Autodesk Fusion 360 part; units mm, degrees
(part 31 of 40)
  spline S99 degree 5 poles (217.8271, 89.2315) (217.8299, 89.2007) (217.8349, 89.1391) (217.8398, 89.0467) (217.8417, 88.9234) (217.8376, 88.769) (217.8289, 88.6144) (217.8174, 88.4597) (217.8043, 88.305) (217.7903, 88.1502) (217.7751, 87.9955) (217.7585, 87.8407) (217.74, 87.686) (217.7191, 87.5312) (217.6961, 87.3765) (217.671, 87.2218) (217.6441, 87.0671) (217.6158, 86.9125) (217.5862, 86.7579) (217.5553, 86.6034) (217.5233, 86.4489) (217.4899, 86.2945) (217.4552, 86.1402) (217.4191, 85.986) (217.3817, 85.8318) (217.3429, 85.6778) (217.3029, 85.5238) (217.2617, 85.3699) (217.2193, 85.2161) (217.1759, 85.0624) (217.1313, 84.9088) (217.0856, 84.7553) (217.0388, 84.602) (216.9909, 84.4487) (216.9419, 84.2956) (216.8919, 84.1426) (216.8407, 83.9897) (216.7886, 83.8369) (216.7355, 83.6842) (216.6813, 83.5317) (216.6262, 83.3794) (216.57, 83.2271) (216.513, 83.075) (216.4549, 82.923) (216.3959, 82.7712) (216.3359, 82.6196) (216.275, 82.468) (216.2132, 82.3167) (216.1505, 82.1655) (216.0868, 82.0144) (216.0223, 81.8635) (215.9569, 81.7128) (215.8905, 81.5622) (215.8233, 81.4118) (215.7553, 81.2616) (215.6863, 81.1115) (215.6166, 80.9616) (215.5459, 80.8119) (215.4745, 80.6624) (215.4021, 80.513) (215.329, 80.3638) (215.255, 80.2148) (215.1802, 80.066) (215.1046, 79.9174) (215.0282, 79.7689) (214.951, 79.6207) (214.873, 79.4726) (214.7942, 79.3248) (214.7146, 79.1771) (214.6343, 79.0297) (214.5531, 78.8824) (214.4876, 78.7648) (214.4381, 78.6766) (214.4049, 78.6179) (214.3883, 78.5885) knots 0 0 0 0 0 0 0.01428571 0.02857143 0.04285714 0.05714286 0.07142857 0.08571429 0.1 0.11428571 0.12857143 0.14285714 0.15714286 0.17142857 0.18571429 0.2 0.21428571 0.22857143 0.24285714 0.25714286 0.27142857 0.28571429 0.3 0.31428571 0.32857143 0.34285714 0.35714286 0.37142857 0.38571429 0.4 0.41428571 0.42857143 0.44285714 0.45714286 0.47142857 0.48571429 0.5 0.51428571 0.52857143 0.54285714 0.55714286 0.57142857 0.58571429 0.6 0.61428571 0.62857143 0.64285714 0.65714286 0.67142857 0.68571429 0.7 0.71428571 0.72857143 0.74285714 0.75714286 0.77142857 0.78571429 0.8 0.81428571 0.82857143 0.84285714 0.85714286 0.87142857 0.88571429 0.9 0.91428571 0.92857143 0.94285714 0.95714286 0.97142857 0.98571429 1 1 1 1 1 1
  line L7434 (217.8271, 89.2315) -> (217.8299, 89.2007) construction
  line L7435 (217.8299, 89.2007) -> (217.8349, 89.1391) construction
  line L7436 (217.8349, 89.1391) -> (217.8398, 89.0467) construction
  line L7437 (217.8398, 89.0467) -> (217.8417, 88.9234) construction
  line L7438 (217.8417, 88.9234) -> (217.8376, 88.769) construction
  line L7439 (217.8376, 88.769) -> (217.8289, 88.6144) construction
  line L7440 (217.8289, 88.6144) -> (217.8174, 88.4597) construction
  line L7441 (217.8174, 88.4597) -> (217.8043, 88.305) construction
  line L7442 (217.8043, 88.305) -> (217.7903, 88.1502) construction
  line L7443 (217.7903, 88.1502) -> (217.7751, 87.9955) construction
  line L7444 (217.7751, 87.9955) -> (217.7585, 87.8407) construction
  line L7445 (217.7585, 87.8407) -> (217.74, 87.686) construction
  line L7446 (217.74, 87.686) -> (217.7191, 87.5312) construction
  line L7447 (217.7191, 87.5312) -> (217.6961, 87.3765) construction
  line L7448 (217.6961, 87.3765) -> (217.671, 87.2218) construction
  line L7449 (217.671, 87.2218) -> (217.6441, 87.0671) construction
  line L7450 (217.6441, 87.0671) -> (217.6158, 86.9125) construction
  line L7451 (217.6158, 86.9125) -> (217.5862, 86.7579) construction
  line L7452 (217.5862, 86.7579) -> (217.5553, 86.6034) construction
  line L7453 (217.5553, 86.6034) -> (217.5233, 86.4489) construction
  line L7454 (217.5233, 86.4489) -> (217.4899, 86.2945) construction
  line L7455 (217.4899, 86.2945) -> (217.4552, 86.1402) construction
  line L7456 (217.4552, 86.1402) -> (217.4191, 85.986) construction
  line L7457 (217.4191, 85.986) -> (217.3817, 85.8318) construction
  line L7458 (217.3817, 85.8318) -> (217.3429, 85.6778) construction
  line L7459 (217.3429, 85.6778) -> (217.3029, 85.5238) construction
  line L7460 (217.3029, 85.5238) -> (217.2617, 85.3699) construction
  line L7461 (217.2617, 85.3699) -> (217.2193, 85.2161) construction
  line L7462 (217.2193, 85.2161) -> (217.1759, 85.0624) construction
  line L7463 (217.1759, 85.0624) -> (217.1313, 84.9088) construction
  line L7464 (217.1313, 84.9088) -> (217.0856, 84.7553) construction
  line L7465 (217.0856, 84.7553) -> (217.0388, 84.602) construction
  line L7466 (217.0388, 84.602) -> (216.9909, 84.4487) construction
  line L7467 (216.9909, 84.4487) -> (216.9419, 84.2956) construction
  line L7468 (216.9419, 84.2956) -> (216.8919, 84.1426) construction
  line L7469 (216.8919, 84.1426) -> (216.8407, 83.9897) construction
  line L7470 (216.8407, 83.9897) -> (216.7886, 83.8369) construction
  line L7471 (216.7886, 83.8369) -> (216.7355, 83.6842) construction
  line L7472 (216.7355, 83.6842) -> (216.6813, 83.5317) construction
  line L7473 (216.6813, 83.5317) -> (216.6262, 83.3794) construction
  line L7474 (216.6262, 83.3794) -> (216.57, 83.2271) construction
  line L7475 (216.57, 83.2271) -> (216.513, 83.075) construction
  line L7476 (216.513, 83.075) -> (216.4549, 82.923) construction
  line L7477 (216.4549, 82.923) -> (216.3959, 82.7712) construction
  line L7478 (216.3959, 82.7712) -> (216.3359, 82.6196) construction
  line L7479 (216.3359, 82.6196) -> (216.275, 82.468) construction
  line L7480 (216.275, 82.468) -> (216.2132, 82.3167) construction
  line L7481 (216.2132, 82.3167) -> (216.1505, 82.1655) construction
  line L7482 (216.1505, 82.1655) -> (216.0868, 82.0144) construction
  line L7483 (216.0868, 82.0144) -> (216.0223, 81.8635) construction
  line L7484 (216.0223, 81.8635) -> (215.9569, 81.7128) construction
  line L7485 (215.9569, 81.7128) -> (215.8905, 81.5622) construction
  line L7486 (215.8905, 81.5622) -> (215.8233, 81.4118) construction
  line L7487 (215.8233, 81.4118) -> (215.7553, 81.2616) construction
  line L7488 (215.7553, 81.2616) -> (215.6863, 81.1115) construction
  line L7489 (215.6863, 81.1115) -> (215.6166, 80.9616) construction
  line L7490 (215.6166, 80.9616) -> (215.5459, 80.8119) construction
  line L7491 (215.5459, 80.8119) -> (215.4745, 80.6624) construction
  line L7492 (215.4745, 80.6624) -> (215.4021, 80.513) construction
  line L7493 (215.4021, 80.513) -> (215.329, 80.3638) construction
  line L7494 (215.329, 80.3638) -> (215.255, 80.2148) construction
  line L7495 (215.255, 80.2148) -> (215.1802, 80.066) construction
  line L7496 (215.1802, 80.066) -> (215.1046, 79.9174) construction
  line L7497 (215.1046, 79.9174) -> (215.0282, 79.7689) construction
  line L7498 (215.0282, 79.7689) -> (214.951, 79.6207) construction
  line L7499 (214.951, 79.6207) -> (214.873, 79.4726) construction
  line L7500 (214.873, 79.4726) -> (214.7942, 79.3248) construction
  line L7501 (214.7942, 79.3248) -> (214.7146, 79.1771) construction
  line L7502 (214.7146, 79.1771) -> (214.6343, 79.0297) construction
  line L7503 (214.6343, 79.0297) -> (214.5531, 78.8824) construction
  line L7504 (214.5531, 78.8824) -> (214.4876, 78.7648) construction
  line L7505 (214.4876, 78.7648) -> (214.4381, 78.6766) construction
  line L7506 (214.4381, 78.6766) -> (214.4049, 78.6179) construction
  line L7507 (214.4049, 78.6179) -> (214.3883, 78.5885) construction
  spline S100 degree 5 poles (257.9473, 109.6737) (257.9705, 109.6533) (258.0174, 109.6132) (258.0893, 109.5549) (258.188, 109.4808) (258.3153, 109.3934) (258.4455, 109.3096) (258.5774, 109.228) (258.7102, 109.1476) (258.8437, 109.068) (258.9778, 108.9893) (259.1127, 108.9117) (259.2488, 108.8358) (259.3863, 108.7617) (259.525, 108.6894) (259.6649, 108.6187) (259.8058, 108.5496) (259.9476, 108.4816) (260.0901, 108.4147) (260.2332, 108.3488) (260.377, 108.284) (260.5215, 108.2202) (260.6667, 108.1576) (260.8127, 108.0961) (260.9594, 108.0358) (261.1069, 107.9766) (261.255, 107.9185) (261.4037, 107.8614) (261.553, 107.8053) (261.7029, 107.7501) (261.8534, 107.6959) (262.0044, 107.6426) (262.156, 107.5903) (262.3081, 107.539) (262.4608, 107.4886) (262.614, 107.4392) (262.7678, 107.3906) (262.922, 107.343) (263.0767, 107.2963) (263.2319, 107.2505) (263.3876, 107.2055) (263.5438, 107.1614) (263.7004, 107.1182) (263.8575, 107.0759) (264.015, 107.0344) (264.1729, 106.9937) (264.3313, 106.9539) (264.4901, 106.915) (264.6493, 106.8769) (264.8089, 106.8396) (264.9689, 106.8031) (265.1293, 106.7674) (265.2901, 106.7326) (265.4513, 106.6985) (265.6129, 106.6653) (265.7748, 106.6328) (265.9371, 106.6012) (266.0997, 106.5703) (266.2627, 106.5403) (266.426, 106.511) (266.5897, 106.4825) (266.7537, 106.4547) (266.9181, 106.4277) (267.0828, 106.4016) (267.2478, 106.3761) (267.4131, 106.3514) (267.5787, 106.3275) (267.7446, 106.3044) (267.9109, 106.282) (268.0774, 106.2603) (268.2442, 106.2394) (268.3779, 106.2233) (268.4783, 106.2115) (268.5453, 106.2038) (268.5789, 106.2) knots 0 0 0 0 0 0 0.01428571 0.02857143 0.04285714 0.05714286 0.07142857 0.08571429 0.1 0.11428571 0.12857143 0.14285714 0.15714286 0.17142857 0.18571429 0.2 0.21428571 0.22857143 0.24285714 0.25714286 0.27142857 0.28571429 0.3 0.31428571 0.32857143 0.34285714 0.35714286 0.37142857 0.38571429 0.4 0.41428571 0.42857143 0.44285714 0.45714286 0.47142857 0.48571429 0.5 0.51428571 0.52857143 0.54285714 0.55714286 0.57142857 0.58571429 0.6 0.61428571 0.62857143 0.64285714 0.65714286 0.67142857 0.68571429 0.7 0.71428571 0.72857143 0.74285714 0.75714286 0.77142857 0.78571429 0.8 0.81428571 0.82857143 0.84285714 0.85714286 0.87142857 0.88571429 0.9 0.91428571 0.92857143 0.94285714 0.95714286 0.97142857 0.98571429 1 1 1 1 1 1
  line L7508 (257.9473, 109.6737) -> (257.9705, 109.6533) construction
  line L7509 (257.9705, 109.6533) -> (258.0174, 109.6132) construction
  line L7510 (258.0174, 109.6132) -> (258.0893, 109.5549) construction
  line L7511 (258.0893, 109.5549) -> (258.188, 109.4808) construction
  line L7512 (258.188, 109.4808) -> (258.3153, 109.3934) construction
  line L7513 (258.3153, 109.3934) -> (258.4455, 109.3096) construction
  line L7514 (258.4455, 109.3096) -> (258.5774, 109.228) construction
  line L7515 (258.5774, 109.228) -> (258.7102, 109.1476) construction
  line L7516 (258.7102, 109.1476) -> (258.8437, 109.068) construction
  line L7517 (258.8437, 109.068) -> (258.9778, 108.9893) construction
  line L7518 (258.9778, 108.9893) -> (259.1127, 108.9117) construction
  line L7519 (259.1127, 108.9117) -> (259.2488, 108.8358) construction
  line L7520 (259.2488, 108.8358) -> (259.3863, 108.7617) construction
  line L7521 (259.3863, 108.7617) -> (259.525, 108.6894) construction
  line L7522 (259.525, 108.6894) -> (259.6649, 108.6187) construction
  line L7523 (259.6649, 108.6187) -> (259.8058, 108.5496) construction
  line L7524 (259.8058, 108.5496) -> (259.9476, 108.4816) construction
  line L7525 (259.9476, 108.4816) -> (260.0901, 108.4147) construction
  line L7526 (260.0901, 108.4147) -> (260.2332, 108.3488) construction
  line L7527 (260.2332, 108.3488) -> (260.377, 108.284) construction
  line L7528 (260.377, 108.284) -> (260.5215, 108.2202) construction
  line L7529 (260.5215, 108.2202) -> (260.6667, 108.1576) construction
  line L7530 (260.6667, 108.1576) -> (260.8127, 108.0961) construction
  line L7531 (260.8127, 108.0961) -> (260.9594, 108.0358) construction
  line L7532 (260.9594, 108.0358) -> (261.1069, 107.9766) construction
  line L7533 (261.1069, 107.9766) -> (261.255, 107.9185) construction
  line L7534 (261.255, 107.9185) -> (261.4037, 107.8614) construction
  line L7535 (261.4037, 107.8614) -> (261.553, 107.8053) construction
  line L7536 (261.553, 107.8053) -> (261.7029, 107.7501) construction
  line L7537 (261.7029, 107.7501) -> (261.8534, 107.6959) construction
  line L7538 (261.8534, 107.6959) -> (262.0044, 107.6426) construction
  line L7539 (262.0044, 107.6426) -> (262.156, 107.5903) construction
  line L7540 (262.156, 107.5903) -> (262.3081, 107.539) construction
  line L7541 (262.3081, 107.539) -> (262.4608, 107.4886) construction
  line L7542 (262.4608, 107.4886) -> (262.614, 107.4392) construction
  line L7543 (262.614, 107.4392) -> (262.7678, 107.3906) construction
  line L7544 (262.7678, 107.3906) -> (262.922, 107.343) construction
  line L7545 (262.922, 107.343) -> (263.0767, 107.2963) construction
  line L7546 (263.0767, 107.2963) -> (263.2319, 107.2505) construction
  line L7547 (263.2319, 107.2505) -> (263.3876, 107.2055) construction
  line L7548 (263.3876, 107.2055) -> (263.5438, 107.1614) construction
  line L7549 (263.5438, 107.1614) -> (263.7004, 107.1182) construction
  line L7550 (263.7004, 107.1182) -> (263.8575, 107.0759) construction
  line L7551 (263.8575, 107.0759) -> (264.015, 107.0344) construction
  line L7552 (264.015, 107.0344) -> (264.1729, 106.9937) construction
  line L7553 (264.1729, 106.9937) -> (264.3313, 106.9539) construction
  line L7554 (264.3313, 106.9539) -> (264.4901, 106.915) construction
  line L7555 (264.4901, 106.915) -> (264.6493, 106.8769) construction
  line L7556 (264.6493, 106.8769) -> (264.8089, 106.8396) construction
  line L7557 (264.8089, 106.8396) -> (264.9689, 106.8031) construction
  line L7558 (264.9689, 106.8031) -> (265.1293, 106.7674) construction
  line L7559 (265.1293, 106.7674) -> (265.2901, 106.7326) construction
  line L7560 (265.2901, 106.7326) -> (265.4513, 106.6985) construction
  line L7561 (265.4513, 106.6985) -> (265.6129, 106.6653) construction
  line L7562 (265.6129, 106.6653) -> (265.7748, 106.6328) construction
  line L7563 (265.7748, 106.6328) -> (265.9371, 106.6012) construction
  line L7564 (265.9371, 106.6012) -> (266.0997, 106.5703) construction
  line L7565 (266.0997, 106.5703) -> (266.2627, 106.5403) construction
  line L7566 (266.2627, 106.5403) -> (266.426, 106.511) construction
  line L7567 (266.426, 106.511) -> (266.5897, 106.4825) construction
  line L7568 (266.5897, 106.4825) -> (266.7537, 106.4547) construction
  line L7569 (266.7537, 106.4547) -> (266.9181, 106.4277) construction
  line L7570 (266.9181, 106.4277) -> (267.0828, 106.4016) construction
  line L7571 (267.0828, 106.4016) -> (267.2478, 106.3761) construction
  line L7572 (267.2478, 106.3761) -> (267.4131, 106.3514) construction
  line L7573 (267.4131, 106.3514) -> (267.5787, 106.3275) construction
  line L7574 (267.5787, 106.3275) -> (267.7446, 106.3044) construction
  line L7575 (267.7446, 106.3044) -> (267.9109, 106.282) construction
  line L7576 (267.9109, 106.282) -> (268.0774, 106.2603) construction
  line L7577 (268.0774, 106.2603) -> (268.2442, 106.2394) construction
  line L7578 (268.2442, 106.2394) -> (268.3779, 106.2233) construction
  line L7579 (268.3779, 106.2233) -> (268.4783, 106.2115) construction
  line L7580 (268.4783, 106.2115) -> (268.5453, 106.2038) construction
  line L7581 (268.5453, 106.2038) -> (268.5789, 106.2) construction
  arc A189 (268.5789, 106.2) -> (271.2313, 109.8508) centre (212.132, 150) ccw
  spline S101 degree 5 poles (171.8057, 104.1847) (171.7853, 104.1615) (171.7452, 104.1146) (171.6869, 104.0427) (171.6128, 103.944) (171.5254, 103.8167) (171.4416, 103.6865) (171.36, 103.5546) (171.2796, 103.4218) (171.2, 103.2883) (171.1213, 103.1542) (171.0437, 103.0193) (170.9678, 102.8832) (170.8937, 102.7457) (170.8214, 102.607) (170.7507, 102.4671) (170.6816, 102.3262) (170.6136, 102.1844) (170.5467, 102.0419) (170.4808, 101.8988) (170.416, 101.755) (170.3522, 101.6105) (170.2896, 101.4653) (170.2281, 101.3193) (170.1678, 101.1726) (170.1086, 101.0251) (170.0505, 100.877) (169.9934, 100.7283) (169.9373, 100.579) (169.8821, 100.4291) (169.8279, 100.2786) (169.7746, 100.1276) (169.7223, 99.976) (169.671, 99.8239) (169.6206, 99.6712) (169.5712, 99.518) (169.5226, 99.3642) (169.475, 99.21) (169.4283, 99.0553) (169.3825, 98.9001) (169.3375, 98.7444) (169.2934, 98.5882) (169.2502, 98.4316) (169.2079, 98.2745) (169.1664, 98.117) (169.1257, 97.9591) (169.0859, 97.8007) (169.047, 97.6419) (169.0089, 97.4827) (168.9716, 97.3231) (168.9351, 97.1631) (168.8994, 97.0027) (168.8646, 96.8419) (168.8305, 96.6807) (168.7973, 96.5191) (168.7648, 96.3572) (168.7332, 96.1949) (168.7023, 96.0323) (168.6723, 95.8693) (168.643, 95.706) (168.6145, 95.5423) (168.5867, 95.3783) (168.5597, 95.2139) (168.5336, 95.0492) (168.5081, 94.8842) (168.4834, 94.7189) (168.4595, 94.5533) (168.4364, 94.3874) (168.414, 94.2211) (168.3923, 94.0546) (168.3714, 93.8878) (168.3553, 93.7541) (168.3435, 93.6537) (168.3358, 93.5867) (168.332, 93.5531) knots 0 0 0 0 0 0 0.01428571 0.02857143 0.04285714 0.05714286 0.07142857 0.08571429 0.1 0.11428571 0.12857143 0.14285714 0.15714286 0.17142857 0.18571429 0.2 0.21428571 0.22857143 0.24285714 0.25714286 0.27142857 0.28571429 0.3 0.31428571 0.32857143 0.34285714 0.35714286 0.37142857 0.38571429 0.4 0.41428571 0.42857143 0.44285714 0.45714286 0.47142857 0.48571429 0.5 0.51428571 0.52857143 0.54285714 0.55714286 0.57142857 0.58571429 0.6 0.61428571 0.62857143 0.64285714 0.65714286 0.67142857 0.68571429 0.7 0.71428571 0.72857143 0.74285714 0.75714286 0.77142857 0.78571429 0.8 0.81428571 0.82857143 0.84285714 0.85714286 0.87142857 0.88571429 0.9 0.91428571 0.92857143 0.94285714 0.95714286 0.97142857 0.98571429 1 1 1 1 1 1
  line L7582 (171.8057, 104.1847) -> (171.7853, 104.1615) construction
  line L7583 (171.7853, 104.1615) -> (171.7452, 104.1146) construction
  line L7584 (171.7452, 104.1146) -> (171.6869, 104.0427) construction
  line L7585 (171.6869, 104.0427) -> (171.6128, 103.944) construction
  line L7586 (171.6128, 103.944) -> (171.5254, 103.8167) construction
  line L7587 (171.5254, 103.8167) -> (171.4416, 103.6865) construction
  line L7588 (171.4416, 103.6865) -> (171.36, 103.5546) construction
  line L7589 (171.36, 103.5546) -> (171.2796, 103.4218) construction
  line L7590 (171.2796, 103.4218) -> (171.2, 103.2883) construction
  line L7591 (171.2, 103.2883) -> (171.1213, 103.1542) construction
  line L7592 (171.1213, 103.1542) -> (171.0437, 103.0193) construction
  line L7593 (171.0437, 103.0193) -> (170.9678, 102.8832) construction
  line L7594 (170.9678, 102.8832) -> (170.8937, 102.7457) construction
  line L7595 (170.8937, 102.7457) -> (170.8214, 102.607) construction
  line L7596 (170.8214, 102.607) -> (170.7507, 102.4671) construction
  line L7597 (170.7507, 102.4671) -> (170.6816, 102.3262) construction
  line L7598 (170.6816, 102.3262) -> (170.6136, 102.1844) construction
  line L7599 (170.6136, 102.1844) -> (170.5467, 102.0419) construction
  line L7600 (170.5467, 102.0419) -> (170.4808, 101.8988) construction
  line L7601 (170.4808, 101.8988) -> (170.416, 101.755) construction
  line L7602 (170.416, 101.755) -> (170.3522, 101.6105) construction
  line L7603 (170.3522, 101.6105) -> (170.2896, 101.4653) construction
  line L7604 (170.2896, 101.4653) -> (170.2281, 101.3193) construction
  line L7605 (170.2281, 101.3193) -> (170.1678, 101.1726) construction
  line L7606 (170.1678, 101.1726) -> (170.1086, 101.0251) construction
  line L7607 (170.1086, 101.0251) -> (170.0505, 100.877) construction
  line L7608 (170.0505, 100.877) -> (169.9934, 100.7283) construction
  line L7609 (169.9934, 100.7283) -> (169.9373, 100.579) construction
  line L7610 (169.9373, 100.579) -> (169.8821, 100.4291) construction
  line L7611 (169.8821, 100.4291) -> (169.8279, 100.2786) construction
  line L7612 (169.8279, 100.2786) -> (169.7746, 100.1276) construction
  line L7613 (169.7746, 100.1276) -> (169.7223, 99.976) construction
  line L7614 (169.7223, 99.976) -> (169.671, 99.8239) construction
  line L7615 (169.671, 99.8239) -> (169.6206, 99.6712) construction
  line L7616 (169.6206, 99.6712) -> (169.5712, 99.518) construction
  line L7617 (169.5712, 99.518) -> (169.5226, 99.3642) construction
  line L7618 (169.5226, 99.3642) -> (169.475, 99.21) construction
  line L7619 (169.475, 99.21) -> (169.4283, 99.0553) construction
  line L7620 (169.4283, 99.0553) -> (169.3825, 98.9001) construction
  line L7621 (169.3825, 98.9001) -> (169.3375, 98.7444) construction
  line L7622 (169.3375, 98.7444) -> (169.2934, 98.5882) construction
  line L7623 (169.2934, 98.5882) -> (169.2502, 98.4316) construction
  line L7624 (169.2502, 98.4316) -> (169.2079, 98.2745) construction
  line L7625 (169.2079, 98.2745) -> (169.1664, 98.117) construction
  line L7626 (169.1664, 98.117) -> (169.1257, 97.9591) construction
  line L7627 (169.1257, 97.9591) -> (169.0859, 97.8007) construction
  line L7628 (169.0859, 97.8007) -> (169.047, 97.6419) construction
  line L7629 (169.047, 97.6419) -> (169.0089, 97.4827) construction
  line L7630 (169.0089, 97.4827) -> (168.9716, 97.3231) construction
  line L7631 (168.9716, 97.3231) -> (168.9351, 97.1631) construction
  line L7632 (168.9351, 97.1631) -> (168.8994, 97.0027) construction
  line L7633 (168.8994, 97.0027) -> (168.8646, 96.8419) construction
  line L7634 (168.8646, 96.8419) -> (168.8305, 96.6807) construction
  line L7635 (168.8305, 96.6807) -> (168.7973, 96.5191) construction
  line L7636 (168.7973, 96.5191) -> (168.7648, 96.3572) construction
  line L7637 (168.7648, 96.3572) -> (168.7332, 96.1949) construction
  line L7638 (168.7332, 96.1949) -> (168.7023, 96.0323) construction
  line L7639 (168.7023, 96.0323) -> (168.6723, 95.8693) construction
  line L7640 (168.6723, 95.8693) -> (168.643, 95.706) construction
  line L7641 (168.643, 95.706) -> (168.6145, 95.5423) construction
  line L7642 (168.6145, 95.5423) -> (168.5867, 95.3783) construction
  line L7643 (168.5867, 95.3783) -> (168.5597, 95.2139) construction
  line L7644 (168.5597, 95.2139) -> (168.5336, 95.0492) construction
  line L7645 (168.5336, 95.0492) -> (168.5081, 94.8842) construction
  line L7646 (168.5081, 94.8842) -> (168.4834, 94.7189) construction
  line L7647 (168.4834, 94.7189) -> (168.4595, 94.5533) construction
  line L7648 (168.4595, 94.5533) -> (168.4364, 94.3874) construction
  line L7649 (168.4364, 94.3874) -> (168.414, 94.2211) construction
  line L7650 (168.414, 94.2211) -> (168.3923, 94.0546) construction
  line L7651 (168.3923, 94.0546) -> (168.3714, 93.8878) construction
  line L7652 (168.3714, 93.8878) -> (168.3553, 93.7541) construction
  line L7653 (168.3553, 93.7541) -> (168.3435, 93.6537) construction
  line L7654 (168.3435, 93.6537) -> (168.3358, 93.5867) construction
  line L7655 (168.3358, 93.5867) -> (168.332, 93.5531) construction
  spline S102 degree 5 poles (225.4942, 209.5542) (225.501, 209.5843) (225.5153, 209.6444) (225.5391, 209.7338) (225.5755, 209.8517) (225.6271, 209.9973) (225.6831, 210.1416) (225.7419, 210.2852) (225.8021, 210.4283) (225.8633, 210.5711) (225.9255, 210.7136) (225.9891, 210.8557) (226.0546, 210.9971) (226.1222, 211.1379) (226.192, 211.2779) (226.2636, 211.4173) (226.337, 211.5561) (226.4117, 211.6944) (226.4877, 211.8322) (226.5647, 211.9697) (226.6429, 212.1067) (226.7224, 212.2432) (226.8031, 212.3792) (226.885, 212.5148) (226.9683, 212.6498) (227.0528, 212.7843) (227.1384, 212.9184) (227.2252, 213.052) (227.313, 213.1852) (227.4018, 213.318) (227.4917, 213.4503) (227.5826, 213.5821) (227.6745, 213.7135) (227.7674, 213.8445) (227.8613, 213.975) (227.9562, 214.105) (228.052, 214.2346) (228.1488, 214.3638) (228.2466, 214.4926) (228.3452, 214.6209) (228.4447, 214.7488) (228.5451, 214.8762) (228.6464, 215.0032) (228.7486, 215.1298) (228.8516, 215.256) (228.9555, 215.3817) (229.0603, 215.507) (229.1658, 215.6318) (229.2722, 215.7562) (229.3794, 215.8802) (229.4875, 216.0038) (229.5963, 216.1269) (229.7059, 216.2497) (229.8162, 216.3719) (229.9274, 216.4938) (230.0393, 216.6152) (230.152, 216.7362) (230.2655, 216.8568) (230.3797, 216.9769) (230.4946, 217.0966) (230.6102, 217.2159) (230.7266, 217.3347) (230.8438, 217.4531) (230.9616, 217.5711) (231.0801, 217.6887) (231.1994, 217.8058) (231.3193, 217.9225) (231.4399, 218.0388) (231.5613, 218.1546) (231.6832, 218.27) (231.8059, 218.385) (231.9046, 218.4767) (231.9789, 218.5452) (232.0286, 218.5908) (232.0535, 218.6136) knots 0 0 0 0 0 0 0.01428571 0.02857143 0.04285714 0.05714286 0.07142857 0.08571429 0.1 0.11428571 0.12857143 0.14285714 0.15714286 0.17142857 0.18571429 0.2 0.21428571 0.22857143 0.24285714 0.25714286 0.27142857 0.28571429 0.3 0.31428571 0.32857143 0.34285714 0.35714286 0.37142857 0.38571429 0.4 0.41428571 0.42857143 0.44285714 0.45714286 0.47142857 0.48571429 0.5 0.51428571 0.52857143 0.54285714 0.55714286 0.57142857 0.58571429 0.6 0.61428571 0.62857143 0.64285714 0.65714286 0.67142857 0.68571429 0.7 0.71428571 0.72857143 0.74285714 0.75714286 0.77142857 0.78571429 0.8 0.81428571 0.82857143 0.84285714 0.85714286 0.87142857 0.88571429 0.9 0.91428571 0.92857143 0.94285714 0.95714286 0.97142857 0.98571429 1 1 1 1 1 1
  line L7656 (225.4942, 209.5542) -> (225.501, 209.5843) construction
  line L7657 (225.501, 209.5843) -> (225.5153, 209.6444) construction
  line L7658 (225.5153, 209.6444) -> (225.5391, 209.7338) construction
  line L7659 (225.5391, 209.7338) -> (225.5755, 209.8517) construction
  line L7660 (225.5755, 209.8517) -> (225.6271, 209.9973) construction
  line L7661 (225.6271, 209.9973) -> (225.6831, 210.1416) construction
  line L7662 (225.6831, 210.1416) -> (225.7419, 210.2852) construction
  line L7663 (225.7419, 210.2852) -> (225.8021, 210.4283) construction
  line L7664 (225.8021, 210.4283) -> (225.8633, 210.5711) construction
  line L7665 (225.8633, 210.5711) -> (225.9255, 210.7136) construction
  line L7666 (225.9255, 210.7136) -> (225.9891, 210.8557) construction
  line L7667 (225.9891, 210.8557) -> (226.0546, 210.9971) construction
  line L7668 (226.0546, 210.9971) -> (226.1222, 211.1379) construction
  line L7669 (226.1222, 211.1379) -> (226.192, 211.2779) construction
  line L7670 (226.192, 211.2779) -> (226.2636, 211.4173) construction
  line L7671 (226.2636, 211.4173) -> (226.337, 211.5561) construction
  line L7672 (226.337, 211.5561) -> (226.4117, 211.6944) construction
  line L7673 (226.4117, 211.6944) -> (226.4877, 211.8322) construction
  line L7674 (226.4877, 211.8322) -> (226.5647, 211.9697) construction
  line L7675 (226.5647, 211.9697) -> (226.6429, 212.1067) construction
  line L7676 (226.6429, 212.1067) -> (226.7224, 212.2432) construction
  line L7677 (226.7224, 212.2432) -> (226.8031, 212.3792) construction
  line L7678 (226.8031, 212.3792) -> (226.885, 212.5148) construction
  line L7679 (226.885, 212.5148) -> (226.9683, 212.6498) construction
  line L7680 (226.9683, 212.6498) -> (227.0528, 212.7843) construction
  line L7681 (227.0528, 212.7843) -> (227.1384, 212.9184) construction
  line L7682 (227.1384, 212.9184) -> (227.2252, 213.052) construction
  line L7683 (227.2252, 213.052) -> (227.313, 213.1852) construction
  line L7684 (227.313, 213.1852) -> (227.4018, 213.318) construction
  line L7685 (227.4018, 213.318) -> (227.4917, 213.4503) construction
  line L7686 (227.4917, 213.4503) -> (227.5826, 213.5821) construction
  line L7687 (227.5826, 213.5821) -> (227.6745, 213.7135) construction
  line L7688 (227.6745, 213.7135) -> (227.7674, 213.8445) construction
  line L7689 (227.7674, 213.8445) -> (227.8613, 213.975) construction
  line L7690 (227.8613, 213.975) -> (227.9562, 214.105) construction
  line L7691 (227.9562, 214.105) -> (228.052, 214.2346) construction
  line L7692 (228.052, 214.2346) -> (228.1488, 214.3638) construction
  line L7693 (228.1488, 214.3638) -> (228.2466, 214.4926) construction
  line L7694 (228.2466, 214.4926) -> (228.3452, 214.6209) construction
  line L7695 (228.3452, 214.6209) -> (228.4447, 214.7488) construction
  line L7696 (228.4447, 214.7488) -> (228.5451, 214.8762) construction
  line L7697 (228.5451, 214.8762) -> (228.6464, 215.0032) construction
  line L7698 (228.6464, 215.0032) -> (228.7486, 215.1298) construction
  line L7699 (228.7486, 215.1298) -> (228.8516, 215.256) construction
  line L7700 (228.8516, 215.256) -> (228.9555, 215.3817) construction
  line L7701 (228.9555, 215.3817) -> (229.0603, 215.507) construction
  line L7702 (229.0603, 215.507) -> (229.1658, 215.6318) construction
  line L7703 (229.1658, 215.6318) -> (229.2722, 215.7562) construction
  line L7704 (229.2722, 215.7562) -> (229.3794, 215.8802) construction
  line L7705 (229.3794, 215.8802) -> (229.4875, 216.0038) construction
  line L7706 (229.4875, 216.0038) -> (229.5963, 216.1269) construction
  line L7707 (229.5963, 216.1269) -> (229.7059, 216.2497) construction
  line L7708 (229.7059, 216.2497) -> (229.8162, 216.3719) construction
  line L7709 (229.8162, 216.3719) -> (229.9274, 216.4938) construction
  line L7710 (229.9274, 216.4938) -> (230.0393, 216.6152) construction
  line L7711 (230.0393, 216.6152) -> (230.152, 216.7362) construction
  line L7712 (230.152, 216.7362) -> (230.2655, 216.8568) construction
  line L7713 (230.2655, 216.8568) -> (230.3797, 216.9769) construction
  line L7714 (230.3797, 216.9769) -> (230.4946, 217.0966) construction
  line L7715 (230.4946, 217.0966) -> (230.6102, 217.2159) construction
  line L7716 (230.6102, 217.2159) -> (230.7266, 217.3347) construction
  line L7717 (230.7266, 217.3347) -> (230.8438, 217.4531) construction
  line L7718 (230.8438, 217.4531) -> (230.9616, 217.5711) construction
  line L7719 (230.9616, 217.5711) -> (231.0801, 217.6887) construction
  line L7720 (231.0801, 217.6887) -> (231.1994, 217.8058) construction
  line L7721 (231.1994, 217.8058) -> (231.3193, 217.9225) construction
  line L7722 (231.3193, 217.9225) -> (231.4399, 218.0388) construction
  line L7723 (231.4399, 218.0388) -> (231.5613, 218.1546) construction
  line L7724 (231.5613, 218.1546) -> (231.6832, 218.27) construction
  line L7725 (231.6832, 218.27) -> (231.8059, 218.385) construction
  line L7726 (231.8059, 218.385) -> (231.9046, 218.4767) construction
  line L7727 (231.9046, 218.4767) -> (231.9789, 218.5452) construction
  line L7728 (231.9789, 218.5452) -> (232.0286, 218.5908) construction
  line L7729 (232.0286, 218.5908) -> (232.0535, 218.6136) construction
  arc A190 (171.9828, 209.0993) -> (168.332, 206.4469) centre (212.132, 150) ccw
  arc A191 (143.5184, 130.0785) -> (144.9129, 125.7868) centre (212.132, 150) ccw
  spline S103 degree 5 poles (225.4942, 209.5542) (225.501, 209.5843) (225.5153, 209.6444) (225.5391, 209.7338) (225.5755, 209.8517) (225.6271, 209.9973) (225.6831, 210.1416) (225.7419, 210.2852) (225.8021, 210.4283) (225.8633, 210.5711) (225.9255, 210.7136) (225.9891, 210.8557) (226.0546, 210.9971) (226.1222, 211.1379) (226.192, 211.2779) (226.2636, 211.4173) (226.337, 211.5561) (226.4117, 211.6944) (226.4877, 211.8322) (226.5647, 211.9697) (226.6429, 212.1067) (226.7224, 212.2432) (226.8031, 212.3792) (226.885, 212.5148) (226.9683, 212.6498) (227.0528, 212.7843) (227.1384, 212.9184) (227.2252, 213.052) (227.313, 213.1852) (227.4018, 213.318) (227.4917, 213.4503) (227.5826, 213.5821) (227.6745, 213.7135) (227.7674, 213.8445) (227.8613, 213.975) (227.9562, 214.105) (228.052, 214.2346) (228.1488, 214.3638) (228.2466, 214.4926) (228.3452, 214.6209) (228.4447, 214.7488) (228.5451, 214.8762) (228.6464, 215.0032) (228.7486, 215.1298) (228.8516, 215.256) (228.9555, 215.3817) (229.0603, 215.507) (229.1658, 215.6318) (229.2722, 215.7562) (229.3794, 215.8802) (229.4875, 216.0038) (229.5963, 216.1269) (229.7059, 216.2497) (229.8162, 216.3719) (229.9274, 216.4938) (230.0393, 216.6152) (230.152, 216.7362) (230.2655, 216.8568) (230.3797, 216.9769) (230.4946, 217.0966) (230.6102, 217.2159) (230.7266, 217.3347) (230.8438, 217.4531) (230.9616, 217.5711) (231.0801, 217.6887) (231.1994, 217.8058) (231.3193, 217.9225) (231.4399, 218.0388) (231.5613, 218.1546) (231.6832, 218.27) (231.8059, 218.385) (231.9046, 218.4767) (231.9789, 218.5452) (232.0286, 218.5908) (232.0535, 218.6136) knots 0 0 0 0 0 0 0.01428571 0.02857143 0.04285714 0.05714286 0.07142857 0.08571429 0.1 0.11428571 0.12857143 0.14285714 0.15714286 0.17142857 0.18571429 0.2 0.21428571 0.22857143 0.24285714 0.25714286 0.27142857 0.28571429 0.3 0.31428571 0.32857143 0.34285714 0.35714286 0.37142857 0.38571429 0.4 0.41428571 0.42857143 0.44285714 0.45714286 0.47142857 0.48571429 0.5 0.51428571 0.52857143 0.54285714 0.55714286 0.57142857 0.58571429 0.6 0.61428571 0.62857143 0.64285714 0.65714286 0.67142857 0.68571429 0.7 0.71428571 0.72857143 0.74285714 0.75714286 0.77142857 0.78571429 0.8 0.81428571 0.82857143 0.84285714 0.85714286 0.87142857 0.88571429 0.9 0.91428571 0.92857143 0.94285714 0.95714286 0.97142857 0.98571429 1 1 1 1 1 1
  line L7730 (225.4942, 209.5542) -> (225.501, 209.5843) construction
  line L7731 (225.501, 209.5843) -> (225.5153, 209.6444) construction
  line L7732 (225.5153, 209.6444) -> (225.5391, 209.7338) construction
  line L7733 (225.5391, 209.7338) -> (225.5755, 209.8517) construction
  line L7734 (225.5755, 209.8517) -> (225.6271, 209.9973) construction
  line L7735 (225.6271, 209.9973) -> (225.6831, 210.1416) construction
  line L7736 (225.6831, 210.1416) -> (225.7419, 210.2852) construction
  line L7737 (225.7419, 210.2852) -> (225.8021, 210.4283) construction
  line L7738 (225.8021, 210.4283) -> (225.8633, 210.5711) construction
  line L7739 (225.8633, 210.5711) -> (225.9255, 210.7136) construction
  line L7740 (225.9255, 210.7136) -> (225.9891, 210.8557) construction
  line L7741 (225.9891, 210.8557) -> (226.0546, 210.9971) construction
  line L7742 (226.0546, 210.9971) -> (226.1222, 211.1379) construction
  line L7743 (226.1222, 211.1379) -> (226.192, 211.2779) construction
  line L7744 (226.192, 211.2779) -> (226.2636, 211.4173) construction
  line L7745 (226.2636, 211.4173) -> (226.337, 211.5561) construction
  line L7746 (226.337, 211.5561) -> (226.4117, 211.6944) construction
  line L7747 (226.4117, 211.6944) -> (226.4877, 211.8322) construction
  line L7748 (226.4877, 211.8322) -> (226.5647, 211.9697) construction
  line L7749 (226.5647, 211.9697) -> (226.6429, 212.1067) construction
  line L7750 (226.6429, 212.1067) -> (226.7224, 212.2432) construction
  line L7751 (226.7224, 212.2432) -> (226.8031, 212.3792) construction
  line L7752 (226.8031, 212.3792) -> (226.885, 212.5148) construction
  line L7753 (226.885, 212.5148) -> (226.9683, 212.6498) construction
  line L7754 (226.9683, 212.6498) -> (227.0528, 212.7843) construction
  line L7755 (227.0528, 212.7843) -> (227.1384, 212.9184) construction
  line L7756 (227.1384, 212.9184) -> (227.2252, 213.052) construction
  line L7757 (227.2252, 213.052) -> (227.313, 213.1852) construction
  line L7758 (227.313, 213.1852) -> (227.4018, 213.318) construction
  line L7759 (227.4018, 213.318) -> (227.4917, 213.4503) construction
  line L7760 (227.4917, 213.4503) -> (227.5826, 213.5821) construction
  line L7761 (227.5826, 213.5821) -> (227.6745, 213.7135) construction
  line L7762 (227.6745, 213.7135) -> (227.7674, 213.8445) construction
  line L7763 (227.7674, 213.8445) -> (227.8613, 213.975) construction
  line L7764 (227.8613, 213.975) -> (227.9562, 214.105) construction
  line L7765 (227.9562, 214.105) -> (228.052, 214.2346) construction
  line L7766 (228.052, 214.2346) -> (228.1488, 214.3638) construction
  line L7767 (228.1488, 214.3638) -> (228.2466, 214.4926) construction
  line L7768 (228.2466, 214.4926) -> (228.3452, 214.6209) construction
  line L7769 (228.3452, 214.6209) -> (228.4447, 214.7488) construction
  line L7770 (228.4447, 214.7488) -> (228.5451, 214.8762) construction
  line L7771 (228.5451, 214.8762) -> (228.6464, 215.0032) construction
  line L7772 (228.6464, 215.0032) -> (228.7486, 215.1298) construction
  line L7773 (228.7486, 215.1298) -> (228.8516, 215.256) construction
  line L7774 (228.8516, 215.256) -> (228.9555, 215.3817) construction
  line L7775 (228.9555, 215.3817) -> (229.0603, 215.507) construction
  line L7776 (229.0603, 215.507) -> (229.1658, 215.6318) construction
  line L7777 (229.1658, 215.6318) -> (229.2722, 215.7562) construction
  line L7778 (229.2722, 215.7562) -> (229.3794, 215.8802) construction
  line L7779 (229.3794, 215.8802) -> (229.4875, 216.0038) construction
  line L7780 (229.4875, 216.0038) -> (229.5963, 216.1269) construction
  line L7781 (229.5963, 216.1269) -> (229.7059, 216.2497) construction
  line L7782 (229.7059, 216.2497) -> (229.8162, 216.3719) construction
  line L7783 (229.8162, 216.3719) -> (229.9274, 216.4938) construction
  line L7784 (229.9274, 216.4938) -> (230.0393, 216.6152) construction
  line L7785 (230.0393, 216.6152) -> (230.152, 216.7362) construction
  line L7786 (230.152, 216.7362) -> (230.2655, 216.8568) construction
  line L7787 (230.2655, 216.8568) -> (230.3797, 216.9769) construction
  line L7788 (230.3797, 216.9769) -> (230.4946, 217.0966) construction
  line L7789 (230.4946, 217.0966) -> (230.6102, 217.2159) construction
  line L7790 (230.6102, 217.2159) -> (230.7266, 217.3347) construction
  line L7791 (230.7266, 217.3347) -> (230.8438, 217.4531) construction
  line L7792 (230.8438, 217.4531) -> (230.9616, 217.5711) construction
  line L7793 (230.9616, 217.5711) -> (231.0801, 217.6887) construction
  line L7794 (231.0801, 217.6887) -> (231.1994, 217.8058) construction
  line L7795 (231.1994, 217.8058) -> (231.3193, 217.9225) construction
  line L7796 (231.3193, 217.9225) -> (231.4399, 218.0388) construction
  line L7797 (231.4399, 218.0388) -> (231.5613, 218.1546) construction
  line L7798 (231.5613, 218.1546) -> (231.6832, 218.27) construction
  line L7799 (231.6832, 218.27) -> (231.8059, 218.385) construction
  line L7800 (231.8059, 218.385) -> (231.9046, 218.4767) construction
  line L7801 (231.9046, 218.4767) -> (231.9789, 218.5452) construction
  line L7802 (231.9789, 218.5452) -> (232.0286, 218.5908) construction
  line L7803 (232.0286, 218.5908) -> (232.0535, 218.6136) construction
  arc A192 (155.697, 160.6816) -> (155.1583, 157.2806) centre (212.132, 150) ccw
  spline S104 degree 5 poles (156.0975, 174.1948) (156.0692, 174.2071) (156.0122, 174.2308) (155.9258, 174.264) (155.8091, 174.3039) (155.6609, 174.3478) (155.5112, 174.3873) (155.3606, 174.4241) (155.2094, 174.4595) (155.0579, 174.494) (154.906, 174.5274) (154.7537, 174.5594) (154.6008, 174.5896) (154.4472, 174.6176) (154.2929, 174.6435) (154.138, 174.6674) (153.9826, 174.6897) (153.8268, 174.7105) (153.6706, 174.7301) (153.5141, 174.7485) (153.3573, 174.7658) (153.2002, 174.7818) (153.0427, 174.7965) (152.8849, 174.8098) (152.7267, 174.8218) (152.5682, 174.8325) (152.4094, 174.842) (152.2503, 174.8504) (152.0909, 174.8577) (151.9313, 174.8638) (151.7715, 174.8689) (151.6114, 174.8729) (151.4511, 174.8757) (151.2905, 174.8776) (151.1297, 174.8783) (150.9687, 174.878) (150.8075, 174.8766) (150.6461, 174.8742) (150.4845, 174.8708) (150.3227, 174.8665) (150.1608, 174.8611) (149.9986, 174.8548) (149.8363, 174.8475) (149.6739, 174.8392) (149.5113, 174.83) (149.3485, 174.8199) (149.1856, 174.8088) (149.0225, 174.7967) (148.8593, 174.7838) (148.696, 174.77) (148.5325, 174.7552) (148.3689, 174.7396) (148.2052, 174.723) (148.0414, 174.7056) (147.8775, 174.6873) (147.7135, 174.6681) (147.5494, 174.648) (147.3852, 174.6271) (147.2209, 174.6054) (147.0565, 174.5828) (146.892, 174.5593) (146.7274, 174.535) (146.5628, 174.5098) (146.398, 174.4839) (146.2333, 174.4571) (146.0684, 174.4294) (145.9035, 174.401) (145.7385, 174.3718) (145.5735, 174.3417) (145.4084, 174.3108) (145.2433, 174.2792) (145.1112, 174.2532) (145.0121, 174.2334) (144.946, 174.22) (144.9129, 174.2132) knots 0 0 0 0 0 0 0.01428571 0.02857143 0.04285714 0.05714286 0.07142857 0.08571429 0.1 0.11428571 0.12857143 0.14285714 0.15714286 0.17142857 0.18571429 0.2 0.21428571 0.22857143 0.24285714 0.25714286 0.27142857 0.28571429 0.3 0.31428571 0.32857143 0.34285714 0.35714286 0.37142857 0.38571429 0.4 0.41428571 0.42857143 0.44285714 0.45714286 0.47142857 0.48571429 0.5 0.51428571 0.52857143 0.54285714 0.55714286 0.57142857 0.58571429 0.6 0.61428571 0.62857143 0.64285714 0.65714286 0.67142857 0.68571429 0.7 0.71428571 0.72857143 0.74285714 0.75714286 0.77142857 0.78571429 0.8 0.81428571 0.82857143 0.84285714 0.85714286 0.87142857 0.88571429 0.9 0.91428571 0.92857143 0.94285714 0.95714286 0.97142857 0.98571429 1 1 1 1 1 1
  line L7804 (156.0975, 174.1948) -> (156.0692, 174.2071) construction
  line L7805 (156.0692, 174.2071) -> (156.0122, 174.2308) construction
  line L7806 (156.0122, 174.2308) -> (155.9258, 174.264) construction
  line L7807 (155.9258, 174.264) -> (155.8091, 174.3039) construction
  line L7808 (155.8091, 174.3039) -> (155.6609, 174.3478) construction
  line L7809 (155.6609, 174.3478) -> (155.5112, 174.3873) construction
  line L7810 (155.5112, 174.3873) -> (155.3606, 174.4241) construction
  line L7811 (155.3606, 174.4241) -> (155.2094, 174.4595) construction
  line L7812 (155.2094, 174.4595) -> (155.0579, 174.494) construction
  line L7813 (155.0579, 174.494) -> (154.906, 174.5274) construction
  line L7814 (154.906, 174.5274) -> (154.7537, 174.5594) construction
  line L7815 (154.7537, 174.5594) -> (154.6008, 174.5896) construction
  line L7816 (154.6008, 174.5896) -> (154.4472, 174.6176) construction
  line L7817 (154.4472, 174.6176) -> (154.2929, 174.6435) construction
  line L7818 (154.2929, 174.6435) -> (154.138, 174.6674) construction
  line L7819 (154.138, 174.6674) -> (153.9826, 174.6897) construction
  line L7820 (153.9826, 174.6897) -> (153.8268, 174.7105) construction
  line L7821 (153.8268, 174.7105) -> (153.6706, 174.7301) construction
  line L7822 (153.6706, 174.7301) -> (153.5141, 174.7485) construction
  line L7823 (153.5141, 174.7485) -> (153.3573, 174.7658) construction
  line L7824 (153.3573, 174.7658) -> (153.2002, 174.7818) construction
  line L7825 (153.2002, 174.7818) -> (153.0427, 174.7965) construction
  line L7826 (153.0427, 174.7965) -> (152.8849, 174.8098) construction
  line L7827 (152.8849, 174.8098) -> (152.7267, 174.8218) construction
  line L7828 (152.7267, 174.8218) -> (152.5682, 174.8325) construction
  line L7829 (152.5682, 174.8325) -> (152.4094, 174.842) construction
  line L7830 (152.4094, 174.842) -> (152.2503, 174.8504) construction
  line L7831 (152.2503, 174.8504) -> (152.0909, 174.8577) construction
  line L7832 (152.0909, 174.8577) -> (151.9313, 174.8638) construction
  line L7833 (151.9313, 174.8638) -> (151.7715, 174.8689) construction
  line L7834 (151.7715, 174.8689) -> (151.6114, 174.8729) construction
  line L7835 (151.6114, 174.8729) -> (151.4511, 174.8757) construction
  line L7836 (151.4511, 174.8757) -> (151.2905, 174.8776) construction
  line L7837 (151.2905, 174.8776) -> (151.1297, 174.8783) construction
  line L7838 (151.1297, 174.8783) -> (150.9687, 174.878) construction
  line L7839 (150.9687, 174.878) -> (150.8075, 174.8766) construction
  line L7840 (150.8075, 174.8766) -> (150.6461, 174.8742) construction
  line L7841 (150.6461, 174.8742) -> (150.4845, 174.8708) construction
  line L7842 (150.4845, 174.8708) -> (150.3227, 174.8665) construction
  line L7843 (150.3227, 174.8665) -> (150.1608, 174.8611) construction
  line L7844 (150.1608, 174.8611) -> (149.9986, 174.8548) construction
  line L7845 (149.9986, 174.8548) -> (149.8363, 174.8475) construction
  line L7846 (149.8363, 174.8475) -> (149.6739, 174.8392) construction
  line L7847 (149.6739, 174.8392) -> (149.5113, 174.83) construction
  line L7848 (149.5113, 174.83) -> (149.3485, 174.8199) construction
  line L7849 (149.3485, 174.8199) -> (149.1856, 174.8088) construction
  line L7850 (149.1856, 174.8088) -> (149.0225, 174.7967) construction
  line L7851 (149.0225, 174.7967) -> (148.8593, 174.7838) construction
  line L7852 (148.8593, 174.7838) -> (148.696, 174.77) construction
  line L7853 (148.696, 174.77) -> (148.5325, 174.7552) construction
  line L7854 (148.5325, 174.7552) -> (148.3689, 174.7396) construction
  line L7855 (148.3689, 174.7396) -> (148.2052, 174.723) construction
  line L7856 (148.2052, 174.723) -> (148.0414, 174.7056) construction
  line L7857 (148.0414, 174.7056) -> (147.8775, 174.6873) construction
  line L7858 (147.8775, 174.6873) -> (147.7135, 174.6681) construction
  line L7859 (147.7135, 174.6681) -> (147.5494, 174.648) construction
  line L7860 (147.5494, 174.648) -> (147.3852, 174.6271) construction
  line L7861 (147.3852, 174.6271) -> (147.2209, 174.6054) construction
  line L7862 (147.2209, 174.6054) -> (147.0565, 174.5828) construction
  line L7863 (147.0565, 174.5828) -> (146.892, 174.5593) construction
  line L7864 (146.892, 174.5593) -> (146.7274, 174.535) construction
  line L7865 (146.7274, 174.535) -> (146.5628, 174.5098) construction
  line L7866 (146.5628, 174.5098) -> (146.398, 174.4839) construction
  line L7867 (146.398, 174.4839) -> (146.2333, 174.4571) construction
  line L7868 (146.2333, 174.4571) -> (146.0684, 174.4294) construction
  line L7869 (146.0684, 174.4294) -> (145.9035, 174.401) construction
  line L7870 (145.9035, 174.401) -> (145.7385, 174.3718) construction
  line L7871 (145.7385, 174.3718) -> (145.5735, 174.3417) construction
  line L7872 (145.5735, 174.3417) -> (145.4084, 174.3108) construction
  line L7873 (145.4084, 174.3108) -> (145.2433, 174.2792) construction
  line L7874 (145.2433, 174.2792) -> (145.1112, 174.2532) construction
  line L7875 (145.1112, 174.2532) -> (145.0121, 174.2334) construction
  line L7876 (145.0121, 174.2334) -> (144.946, 174.22) construction
  line L7877 (144.946, 174.22) -> (144.9129, 174.2132) construction
  spline S105 degree 5 poles (271.6862, 136.6378) (271.7163, 136.631) (271.7764, 136.6167) (271.8658, 136.5929) (271.9837, 136.5565) (272.1293, 136.5049) (272.2736, 136.4489) (272.4172, 136.3901) (272.5603, 136.3299) (272.7031, 136.2687) (272.8456, 136.2065) (272.9877, 136.1429) (273.1291, 136.0774) (273.2699, 136.0098) (273.4099, 135.94) (273.5493, 135.8684) (273.6881, 135.795) (273.8264, 135.7203) (273.9642, 135.6443) (274.1017, 135.5673) (274.2387, 135.4891) (274.3752, 135.4096) (274.5112, 135.3289) (274.6468, 135.247) (274.7818, 135.1637) (274.9163, 135.0792) (275.0504, 134.9936) (275.184, 134.9068) (275.3172, 134.819) (275.45, 134.7302) (275.5823, 134.6403) (275.7141, 134.5494) (275.8455, 134.4575) (275.9765, 134.3646) (276.107, 134.2707) (276.237, 134.1758) (276.3666, 134.08) (276.4958, 133.9832) (276.6246, 133.8854) (276.7529, 133.7868) (276.8808, 133.6873) (277.0082, 133.5869) (277.1352, 133.4856) (277.2618, 133.3834) (277.388, 133.2804) (277.5137, 133.1765) (277.639, 133.0717) (277.7638, 132.9662) (277.8882, 132.8598) (278.0122, 132.7526) (278.1358, 132.6445) (278.2589, 132.5357) (278.3817, 132.4261) (278.5039, 132.3158) (278.6258, 132.2046) (278.7472, 132.0927) (278.8682, 131.98) (278.9888, 131.8665) (279.1089, 131.7523) (279.2286, 131.6374) (279.3479, 131.5218) (279.4667, 131.4054) (279.5851, 131.2882) (279.7031, 131.1704) (279.8207, 131.0519) (279.9378, 130.9326) (280.0545, 130.8127) (280.1708, 130.6921) (280.2866, 130.5707) (280.402, 130.4488) (280.517, 130.3261) (280.6087, 130.2274) (280.6772, 130.1531) (280.7228, 130.1034) (280.7456, 130.0785) knots 0 0 0 0 0 0 0.01428571 0.02857143 0.04285714 0.05714286 0.07142857 0.08571429 0.1 0.11428571 0.12857143 0.14285714 0.15714286 0.17142857 0.18571429 0.2 0.21428571 0.22857143 0.24285714 0.25714286 0.27142857 0.28571429 0.3 0.31428571 0.32857143 0.34285714 0.35714286 0.37142857 0.38571429 0.4 0.41428571 0.42857143 0.44285714 0.45714286 0.47142857 0.48571429 0.5 0.51428571 0.52857143 0.54285714 0.55714286 0.57142857 0.58571429 0.6 0.61428571 0.62857143 0.64285714 0.65714286 0.67142857 0.68571429 0.7 0.71428571 0.72857143 0.74285714 0.75714286 0.77142857 0.78571429 0.8 0.81428571 0.82857143 0.84285714 0.85714286 0.87142857 0.88571429 0.9 0.91428571 0.92857143 0.94285714 0.95714286 0.97142857 0.98571429 1 1 1 1 1 1
  line L7878 (271.6862, 136.6378) -> (271.7163, 136.631) construction
  line L7879 (271.7163, 136.631) -> (271.7764, 136.6167) construction
  line L7880 (271.7764, 136.6167) -> (271.8658, 136.5929) construction
  line L7881 (271.8658, 136.5929) -> (271.9837, 136.5565) construction
  line L7882 (271.9837, 136.5565) -> (272.1293, 136.5049) construction
  line L7883 (272.1293, 136.5049) -> (272.2736, 136.4489) construction
  line L7884 (272.2736, 136.4489) -> (272.4172, 136.3901) construction
  line L7885 (272.4172, 136.3901) -> (272.5603, 136.3299) construction
  line L7886 (272.5603, 136.3299) -> (272.7031, 136.2687) construction
  line L7887 (272.7031, 136.2687) -> (272.8456, 136.2065) construction
  line L7888 (272.8456, 136.2065) -> (272.9877, 136.1429) construction
  line L7889 (272.9877, 136.1429) -> (273.1291, 136.0774) construction
  line L7890 (273.1291, 136.0774) -> (273.2699, 136.0098) construction
  line L7891 (273.2699, 136.0098) -> (273.4099, 135.94) construction
  line L7892 (273.4099, 135.94) -> (273.5493, 135.8684) construction
  line L7893 (273.5493, 135.8684) -> (273.6881, 135.795) construction
  line L7894 (273.6881, 135.795) -> (273.8264, 135.7203) construction
  line L7895 (273.8264, 135.7203) -> (273.9642, 135.6443) construction
  line L7896 (273.9642, 135.6443) -> (274.1017, 135.5673) construction
  line L7897 (274.1017, 135.5673) -> (274.2387, 135.4891) construction
  line L7898 (274.2387, 135.4891) -> (274.3752, 135.4096) construction
  line L7899 (274.3752, 135.4096) -> (274.5112, 135.3289) construction
  line L7900 (274.5112, 135.3289) -> (274.6468, 135.247) construction
  line L7901 (274.6468, 135.247) -> (274.7818, 135.1637) construction
  line L7902 (274.7818, 135.1637) -> (274.9163, 135.0792) construction
  line L7903 (274.9163, 135.0792) -> (275.0504, 134.9936) construction
  line L7904 (275.0504, 134.9936) -> (275.184, 134.9068) construction
  line L7905 (275.184, 134.9068) -> (275.3172, 134.819) construction
  line L7906 (275.3172, 134.819) -> (275.45, 134.7302) construction
  line L7907 (275.45, 134.7302) -> (275.5823, 134.6403) construction
  line L7908 (275.5823, 134.6403) -> (275.7141, 134.5494) construction
  line L7909 (275.7141, 134.5494) -> (275.8455, 134.4575) construction
  line L7910 (275.8455, 134.4575) -> (275.9765, 134.3646) construction
  line L7911 (275.9765, 134.3646) -> (276.107, 134.2707) construction
  line L7912 (276.107, 134.2707) -> (276.237, 134.1758) construction